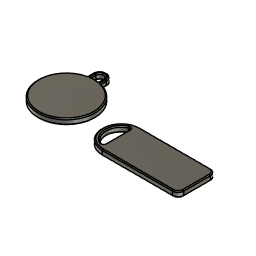
Key Chain template (Autodesk Fusion 360 design; units mm, degrees)
Autodesk Fusion 360 part; units mm, degrees
sketch "Round Keychain" plane through (0, 0, 0) normal (0, 0, 1) x (1, 0, 0)
  circle A0 centre (0, 0) radius 15
  line L0 (3.5, 0) -> (3.5, 17.5)
  arc A1 (3.5, 17.5) -> (-3.5, 17.5) centre (0, 17.5) ccw
  line L1 (-3.5, 17.5) -> (-3.5, 0)
  arc A2 (-3.5, 0) -> (3.5, 0) centre (0, 0) ccw
  line L2 (0, 0) -> (0, 17.5) construction
  line L3 (2, 0) -> (2, 17.5)
  arc A3 (2, 17.5) -> (-2, 17.5) centre (0, 17.5) ccw
  line L4 (-2, 17.5) -> (-2, 0)
  arc A4 (-2, 0) -> (2, 0) centre (0, 0) ccw
  dimension "d1" = 30
  dimension "d2" = 7
  dimension "d3" = 17.5
  dimension "d4" = -1.5
  constraint coincident A0.centre A2.centre
  constraint tangent L0 A1
  constraint tangent A1 L1
  constraint parallel L0 L1
  constraint tangent L1 A2
  constraint tangent L0 A2
  constraint vertical L2
  measures "d1" diameter of A0
  measures "d2" diameter of A1
  measures "d3" distance of A0.centre A1.centre
extrude "Extrude1" add sketch "Round Keychain" along normal blind 3 contours A0 L0 L1 A2 | A0 L0 L1 A2 L3 L4 A4 | A0 L0 A1 L1 L3 A3 L4 | A0 L3 L4 A4 makes body 1
chamfer "Chamfer1" distance 0.5 angle 45 2 faces at (-0.6135, -8.6593, 3) (-0.6135, -8.6593, 0) on bodies 1
sketch "Sketch2" plane through (0, 0, 0) normal (0, 0, 1) x (1, 0, 0)
  line L0 (34.086, 4.7938) -> (71.086, 4.7938)
  line L1 (74.086, 1.7938) -> (74.086, -12.2062)
  line L2 (71.086, -15.2062) -> (34.086, -15.2062)
  line L3 (34.086, 4.7938) -> (34.086, -15.2062)
  arc A0 (34.086, 4.7938) -> (34.086, -15.2062) centre (34.086, -5.2062) ccw
  line L4 (32.086, 1.1184) -> (32.086, -11.5307)
  arc A1 (30.6574, 2.0219) -> (30.6574, -12.4342) centre (34.086, -5.2062) ccw
  arc A2 (32.086, 1.1184) -> (30.6574, 2.0219) centre (31.086, 1.1184) ccw
  arc A3 (30.6574, -12.4342) -> (32.086, -11.5307) centre (31.086, -11.5307) ccw
  arc A4 (74.086, 1.7938) -> (71.086, 4.7938) centre (71.086, 1.7938) ccw
  arc A5 (71.086, -15.2062) -> (74.086, -12.2062) centre (71.086, -12.2062) ccw
  dimension "d10" = 20
  dimension "d13" = 1
  dimension "d14" = 3
  constraint horizontal L0
  constraint vertical L1
  constraint horizontal L2
  constraint perpendicular L2 L3
  constraint concentric A0 A1
  constraint tangent L4 A2
  constraint tangent A1 A2
  constraint tangent L4 A3
  constraint tangent A1 A3
  constraint equal A2 A3
  constraint tangent L0 A4
  constraint tangent L1 A4
  constraint tangent L1 A5
  constraint tangent L2 A5
  constraint equal A4 A5
  measures "d10" diameter of A0
  measures "d13" radius of A2
  measures "d14" radius of A4
extrude "Extrude2" add sketch "Sketch2" along normal blind 3 separate body makes body 2
chamfer "Chamfer2" distance 0.5 angle 45 2 faces at (58.7527, -8.5395, 0) (58.7527, -8.5395, 3) on bodies 2
